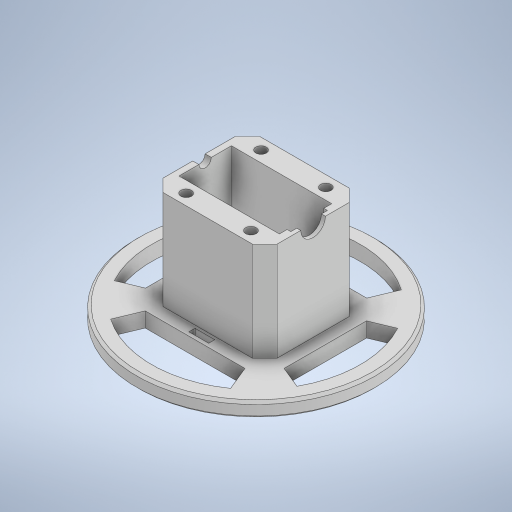
# Autodesk Inventor part: Base_baSECap
Saved by Autodesk Inventor 2023 (Build 270158000, 158)
## iProperties
Created: 2025-02-06
Part Number: Base_baSECap
Material: Generic
Document SubType Name: Modeling
Designer: Swoby
Density: 1 g/cm^3
Appearance: Default
Author: Swoby
Autodesk Inventor part; units mm, degrees
ref_plane "YZ Plane" through (0, 0, 0) normal (1, 0, 0) x (0, 1, 0)
ref_plane "XZ Plane" through (0, 0, 0) normal (0, 1, 0) x (-1, 0, 0)
ref_plane "XY Plane" through (0, 0, 0) normal (0, 0, 1) x (1, 0, 0)
sketch "Sketch1" plane through (0, 0, 0) normal (0, 0, 1) x (1, 0, 0)
  line L0 (0, 3) -> (0, -3)
  line L1 (0, 3) -> (47.2, 3)
  line L2 (48.2, 2) -> (48.2, -2)
  line L3 (47.2, -3) -> (0, -3)
  line L4 (0, 0) -> (48.2, 0) construction
  line L5 (47.2, 3) -> (48.2, 2)
  line L6 (48.2, -2) -> (47.2, -3)
  point P0 (48.2, 3)
  point P1 (48.2, -3)
  dimension "d0" = 96.4
  dimension "d1" = 6
  dimension "d2" = 1
  dimension "d3" = 1
  dimension "d4" = 1
  dimension "d5" = 1
  constraints: 14 end point, 4 point on line, 3 perpendicular, 2 midpoint, 1 horizontal, 1 vertical
  measures "d0" diameter of L2 L0
  measures "d1" distance of point (48.2, 3) point (48.2, -3)
  measures "d2" distance of L1.end point (48.2, 3)
  measures "d3" distance of L2.start point (48.2, 3)
  measures "d4" distance of L2.end point (48.2, -3)
  measures "d5" distance of L3.start point (48.2, -3)
revolve "Revolution1" add sketch "Sketch1" angle 360 about axis through (0, 3, 0) along (0, -1, 0)
sketch "Sketch2" plane through (0, -3, 0) normal (0, -1, 0) x (1, 0, 0)
  circle A0 centre (0, 0) radius 47.2 projected
  line L0 (0, 0) -> (47.2, 0) construction
  line L1 (0, 0) -> (12.9047, -12.9047) construction
  line L2 (0, 0) -> (-12.9047, -12.9047) construction
  arc A1 (11.7375, -14.5288) -> (14.3189, -14.3189) centre (12.9047, -12.9047) ccw
  arc A2 (-14.3189, -14.3189) -> (-11.7375, -14.5288) centre (-12.9047, -12.9047) ccw
  line L3 (4.5962, -4.5962) -> (1.8031, -7.3893) construction
  line L4 (-4.5962, -4.5962) -> (-1.8031, -7.3893) construction
  line L5 (12.9047, -12.9047) -> (14.3189, -14.3189) construction
  line L6 (-12.9047, -12.9047) -> (-14.3189, -14.3189) construction
  line L7 (-1.8031, -7.3893) -> (-11.7375, -14.5288)
  line L8 (1.8031, -7.3893) -> (11.7375, -14.5288)
  arc A3 (1.8031, -7.3893) -> (-1.8031, -7.3893) centre (0, -9.8982) ccw
  line L9 (4.5962, 4.5962) -> (7.3893, 1.8031) construction
  line L10 (7.3893, 1.8031) -> (14.5288, 11.7375)
  line L11 (12.9047, 12.9047) -> (14.3189, 14.3189) construction
  arc A4 (14.5288, 11.7375) -> (14.3189, 14.3189) centre (12.9047, 12.9047) ccw
  arc A5 (7.3893, 1.8031) -> (7.3893, -1.8031) centre (9.8982, 0) ccw
  line L12 (4.5962, -4.5962) -> (7.3893, -1.8031) construction
  line L13 (7.3893, -1.8031) -> (14.5288, -11.7375)
  arc A6 (14.3189, -14.3189) -> (14.5288, -11.7375) centre (12.9047, -12.9047) ccw
  line L14 (12.9047, -12.9047) -> (14.3189, -14.3189) construction
  line L15 (-4.5962, 4.5962) -> (-1.8031, 7.3893) construction
  line L16 (-1.8031, 7.3893) -> (-11.7375, 14.5288)
  line L17 (-12.9047, 12.9047) -> (-14.3189, 14.3189) construction
  arc A7 (-11.7375, 14.5288) -> (-14.3189, 14.3189) centre (-12.9047, 12.9047) ccw
  arc A8 (-1.8031, 7.3893) -> (1.8031, 7.3893) centre (0, 9.8982) ccw
  line L18 (4.5962, 4.5962) -> (1.8031, 7.3893) construction
  line L19 (1.8031, 7.3893) -> (11.7375, 14.5288)
  arc A9 (14.3189, 14.3189) -> (11.7375, 14.5288) centre (12.9047, 12.9047) ccw
  line L20 (12.9047, 12.9047) -> (14.3189, 14.3189) construction
  line L21 (-4.5962, -4.5962) -> (-7.3893, -1.8031) construction
  line L22 (-7.3893, -1.8031) -> (-14.5288, -11.7375)
  line L23 (-12.9047, -12.9047) -> (-14.3189, -14.3189) construction
  arc A10 (-14.5288, -11.7375) -> (-14.3189, -14.3189) centre (-12.9047, -12.9047) ccw
  arc A11 (-7.3893, -1.8031) -> (-7.3893, 1.8031) centre (-9.8982, 0) ccw
  line L24 (-4.5962, 4.5962) -> (-7.3893, 1.8031) construction
  line L25 (-7.3893, 1.8031) -> (-14.5288, 11.7375)
  arc A12 (-14.3189, 14.3189) -> (-14.5288, 11.7375) centre (-12.9047, 12.9047) ccw
  line L26 (-12.9047, 12.9047) -> (-14.3189, 14.3189) construction
  circle A13 centre (0, 0) radius 3.4
  point P0 (0, 0)
  dimension "d7" = 45
  dimension "d8" = 18.25
  dimension "d9" = 18.25
  dimension "d10" = 4
  dimension "d11" = 4
  dimension "d13" = 6.5
  dimension "d14" = 6.5
  dimension "d15" = 3.95
  dimension "d16" = 3.95
  dimension "d19" = 360
  dimension "d68" = 6.8
  constraints: 54 end point, 24 point on circle, 13 centre point, 9 coincident, 3 perpendicular, 3 tangent, 2 collinear, 2 point on line, 1 horizontal, 1 horizontal alignment, 90 other
  measures "d7" angle of L0 L1
  measures "d8" distance of L0.start L1.end
  measures "d9" distance of L0.start L2.end
  measures "d10" diameter of A1
  measures "d11" diameter of A2
  measures "d13" distance from line of point (0, 0) L3
  measures "d14" distance from line of point (0, 0) L4
  measures "d15" distance of L4.start L4.end
  measures "d16" distance of L3.start L3.end
  measures "d68" diameter of A13
extrude "Extrusion1" cut sketch "Sketch2" against normal blind 4 contours L8 A3 L7 A2 A10 L22 A11 L25 A12 A7 L16 A8 L19 A9 A4 L10 A5 L13 A6 A1 | A13
sketch "Sketch3" plane through (0, 1, 0) normal (0, -1, 0) x (1, 0, 0)
  arc A0 (11.7375, -14.5288) -> (14.5288, -11.7375) centre (12.9047, -12.9047) ccw projected
  line L0 (7.3893, -1.8031) -> (14.5288, -11.7375) projected
  arc A1 (7.3893, 1.8031) -> (7.3893, -1.8031) centre (9.8982, 0) ccw projected
  line L1 (14.5288, 11.7375) -> (7.3893, 1.8031) projected
  arc A2 (14.5288, 11.7375) -> (11.7375, 14.5288) centre (12.9047, 12.9047) ccw projected
  line L2 (1.8031, 7.3893) -> (11.7375, 14.5288) projected
  arc A3 (-1.8031, 7.3893) -> (1.8031, 7.3893) centre (0, 9.8982) ccw projected
  line L3 (-11.7375, 14.5288) -> (-1.8031, 7.3893) projected
  arc A4 (-11.7375, 14.5288) -> (-14.5288, 11.7375) centre (-12.9047, 12.9047) ccw projected
  line L4 (-7.3893, 1.8031) -> (-14.5288, 11.7375) projected
  arc A5 (-7.3893, -1.8031) -> (-7.3893, 1.8031) centre (-9.8982, 0) ccw projected
  line L5 (-14.5288, -11.7375) -> (-7.3893, -1.8031) projected
  arc A6 (-14.5288, -11.7375) -> (-11.7375, -14.5288) centre (-12.9047, -12.9047) ccw projected
  line L6 (-1.8031, -7.3893) -> (-11.7375, -14.5288) projected
  arc A7 (1.8031, -7.3893) -> (-1.8031, -7.3893) centre (0, -9.8982) ccw projected
  line L7 (11.7375, -14.5288) -> (1.8031, -7.3893) projected
  circle A8 centre (-12.9047, 12.9047) radius 0.5
  circle A9 centre (-12.9047, -12.9047) radius 0.5
  circle A10 centre (12.9047, -12.9047) radius 0.5
  circle A11 centre (12.9047, 12.9047) radius 0.5
  point P0 (0, 0)
  dimension "d23" = 1
  dimension "d24" = 1
  dimension "d25" = 1
  dimension "d26" = 1
  constraints: 4 centre point, 4 coincident
  measures "d23" diameter of A8
  measures "d24" diameter of A9
  measures "d25" diameter of A10
  measures "d26" diameter of A11
extrude "Extrusion2" cut sketch "Sketch3" against normal blind 6 contours A8 | A9 | A10 | A11
sketch "Sketch4" plane through (0, 3, 0) normal (0, 1, 0) x (1, 0, 0)
  line L0 (20, 10.65) -> (12.5, 10.65)
  line L1 (-20.6, 10.65) -> (-20.6, -10.55)
  line L2 (-20.6, -10.55) -> (8.8, -10.55)
  line L3 (20, -10.55) -> (20, 10.65)
  line L4 (21.5, 7.4) -> (20, 7.4)
  line L5 (20, 7.4) -> (20, 0)
  line L6 (21.5, 0) -> (21.5, 7.4)
  line L7 (23.1, 5) -> (21.5, 5)
  line L8 (21.5, 5) -> (21.5, 0)
  line L9 (20, 0) -> (23.1, 0)
  line L10 (23.1, 0) -> (23.1, 5)
  line L11 (8.8, 10.65) -> (12.5, 10.65)
  line L12 (8.8, -10.55) -> (12.5, -10.55)
  line L13 (-16.7, 10.65) -> (-11.3, 10.65)
  line L14 (-16.7, 10.65) -> (-20.6, 10.65)
  line L15 (-11.3, 10.65) -> (-16.7, 10.65)
  line L16 (12.5, 10.65) -> (12.5, 10.65)
  line L17 (8.8, 10.65) -> (-11.3, 10.65)
  line L18 (12.5, 10.65) -> (8.8, 10.65)
  line L19 (8.8, -10.55) -> (12.5, -10.55)
  line L20 (12.5, -10.55) -> (20, -10.55)
  line L21 (-23.1, 14.65) -> (-23.1, -14.55)
  line L22 (-18.1, 19.65) -> (18.1, 19.65)
  line L23 (23.1, 14.65) -> (23.1, -14.55)
  line L24 (18.1, -19.55) -> (-18.1, -19.55)
  line L25 (-23.1, -14.55) -> (-18.1, -19.55)
  line L26 (18.1, -19.55) -> (23.1, -14.55)
  line L27 (18.1, 19.65) -> (23.1, 14.65)
  line L28 (-18.1, 19.65) -> (-23.1, 14.65)
  line L29 (-23.1, 0) -> (23.1, 0) construction
  line L30 (8.8, 10.65) -> (8.8, -10.55)
  line L31 (12.5, -10.55) -> (12.5, 10.65)
  line L32 (-16.7, 10.65) -> (-16.7, -10.55) construction
  line L33 (-11.3, 10.65) -> (-11.3, -10.55) construction
  point P0 (0, 0)
  point P1 (-23.1, 19.65)
  point P2 (-23.1, -19.55)
  point P3 (-23.1, -2.3384)
  point P4 (23.1, 19.65)
  point P5 (23.1, -19.55)
  point P6 (-16.7, 19.65)
  point P7 (-11.3, 19.65)
  point P8 (0, 0)
  dimension "d29" = 10.65
  dimension "d30" = 1.5
  dimension "d31" = 1.6
  dimension "d32" = 21.2
  dimension "d33" = 40.6
  dimension "d40" = 2.5
  dimension "d41" = 5
  dimension "d47" = 5
  dimension "d48" = 5
  dimension "d49" = 5
  dimension "d50" = 5
  dimension "d51" = 5
  dimension "d52" = 5
  dimension "d53" = 5
  dimension "d54" = 5
  dimension "d57" = 7.4
  dimension "d77" = 3.7
  dimension "d78" = 7.5
  dimension "d79" = 3.9
  dimension "d80" = 5.4
  dimension "d81" = 9
  dimension "d82" = 9
  constraints: 68 end point, 21 parallel, 17 point on line, 12 horizontal, 11 perpendicular, 1 coincident, 1 collinear, 1 midpoint, 1 vertical
  measures "d29" distance from line of L5.end L0
  measures "d30" distance of L4.start L4.end
  measures "d31" distance of L7.start L7.end
  measures "d32" distance of L3.start L0.start
  measures "d33" distance between parallel lines of L3 L1
  measures "d40" distance from line of L1 point (-23.1, -2.338)
  measures "d41" distance between parallel lines of L9 L7
  measures "d47" distance of L21.end point (-23.1, -19.55)
  measures "d48" distance of L24.end point (-23.1, -19.55)
  measures "d49" distance of L24.start point (23.1, -19.55)
  measures "d50" distance of L23.end point (23.1, -19.55)
  measures "d51" distance of L22.end point (23.1, 19.65)
  measures "d52" distance of L23.start point (23.1, 19.65)
  measures "d53" distance of L22.start point (-23.1, 19.65)
  measures "d54" distance of L21.start point (-23.1, 19.65)
  measures "d57" distance between parallel lines of L9 L4
  measures "d77" distance between parallel lines of L30 L31
  measures "d78" distance between parallel lines of L3 L31
  measures "d79" distance between parallel lines of L32 L1
  measures "d80" distance between parallel lines of L33 L32
  measures "d81" distance between parallel lines of L17 L22
  measures "d82" distance between parallel lines of L24 L20
extrude "Extrusion3" add sketch "Sketch4" along normal blind 40
extrude "Extrusion5" cut sketch "Sketch4" against normal blind 30.95 from surface at 40 contours L3 L20 L31 L0 | L31 L12 L30 L11 | L30 L2 L1 L14 L13 L17
sketch "Sketch5" plane through (0, 43, 0) normal (0, 1, 0) x (1, 0, 0)
  line L0 (18.1, 19.65) -> (-18.1, 19.65) projected
  line L1 (-18.1, 19.65) -> (-23.1, 14.65) projected
  line L2 (-23.1, 14.65) -> (-23.1, -14.55) projected
  line L3 (-23.1, -14.55) -> (-18.1, -19.55) projected
  line L4 (-18.1, -19.55) -> (18.1, -19.55) projected
  line L5 (18.1, -19.55) -> (23.1, -14.55) projected
  line L6 (23.1, -14.55) -> (23.1, 14.65) projected
  line L7 (23.1, 14.65) -> (18.1, 19.65) projected
  line L8 (-20.6, 10.65) -> (20, 10.65) projected
  line L9 (20, 10.65) -> (20, -10.55) projected
  line L10 (20, -10.55) -> (-20.6, -10.55) projected
  line L11 (-20.6, -10.55) -> (-20.6, 10.65) projected
  line L12 (20, 7.4) -> (21.5, 7.4)
  line L13 (21.5, 7.4) -> (21.5, 5)
  line L14 (21.5, 5) -> (23.1, 5)
  line L15 (23.1, 5) -> (23.1, 0)
  line L16 (23.1, 0) -> (20, 0)
  line L17 (20, 7.4) -> (20, 0)
  line L18 (-23.1, 0) -> (-20.6, 0)
  line L19 (-20.6, 0) -> (-20.6, 2.5)
  line L20 (-20.6, 2.5) -> (-23.1, 2.5)
  line L21 (-23.1, 2.5) -> (-23.1, 0)
  point P0 (0, 0)
  point P1 (-21.85, 0)
  dimension "d62" = 10
  dimension "d63" = 14.8
  dimension "d64" = 1.5
  dimension "d66" = 5
  constraints: 20 end point, 8 point on line, 4 perpendicular, 2 horizontal, 2 parallel, 1 collinear, 1 midpoint
  measures "d62" diameter of L14 L16
  measures "d63" diameter of L12 L16
  measures "d64" distance of L12.start L12.end
  measures "d66" diameter of L20 point (-21.85, 0)
revolve "Revolution2" cut sketch "Sketch5" angle 360 about axis through (23.1, 43, 0) along (-1, 0, 0) contours L6 L16 L9 L12 L13 L14 | L20 L11 L18 L2
extrude "Extrusion6" cut sketch "Sketch2" against normal through all contours A13
sketch "Sketch6" plane through (0, 43, 0) normal (0, 1, 0) x (1, 0, 0)
  line L0 (21.5, 5) -> (23.1, 5) projected
  line L1 (23.1, 5) -> (23.1, 14.65) projected
  line L2 (23.1, 14.65) -> (18.1, 19.65) projected
  line L3 (18.1, 19.65) -> (-18.1, 19.65) projected
  line L4 (-18.1, 19.65) -> (-23.1, 14.65) projected
  line L5 (-23.1, 14.65) -> (-23.1, 2.5) projected
  line L6 (-23.1, 2.5) -> (-20.6, 2.5) projected
  line L7 (-20.6, 2.5) -> (-20.6, 10.65) projected
  line L8 (-20.6, 10.65) -> (20, 10.65) projected
  line L9 (20, 10.65) -> (20, 7.4) projected
  line L10 (20, 7.4) -> (21.5, 7.4) projected
  line L11 (21.5, 7.4) -> (21.5, 5) projected
  line L12 (23.1, -5) -> (21.5, -5) projected
  line L13 (21.5, -5) -> (21.5, -7.4) projected
  line L14 (21.5, -7.4) -> (20, -7.4) projected
  line L15 (20, -7.4) -> (20, -10.55) projected
  line L16 (20, -10.55) -> (-20.6, -10.55) projected
  line L17 (-20.6, -10.55) -> (-20.6, -2.5) projected
  line L18 (-20.6, -2.5) -> (-23.1, -2.5) projected
  line L19 (-23.1, -2.5) -> (-23.1, -14.55) projected
  line L20 (-23.1, -14.55) -> (-18.1, -19.55) projected
  line L21 (-18.1, -19.55) -> (18.1, -19.55) projected
  line L22 (18.1, -19.55) -> (23.1, -14.55) projected
  line L23 (23.1, -14.55) -> (23.1, -5) projected
  line L24 (-18.1, 19.65) -> (-18.1, 10.65) construction
  line L25 (-18.1, 15.15) -> (0, 15.15) construction
  circle A0 centre (-13.1, 15.15) radius 2.15
  line L26 (0, 19.65) -> (0, 0) construction
  circle A1 centre (0, 0) radius 3.4 projected
  line L27 (0, 0) -> (-23.1, 0) construction
  circle A2 centre (13.1, 15.15) radius 2.15
  line L28 (0, 0) -> (23.1, 0) construction
  circle A3 centre (-13.1, -15.15) radius 2.15
  circle A4 centre (13.1, -15.15) radius 2.15
  dimension "d83" = 4.3
  dimension "d84" = 5
  constraints: 10 end point, 4 centre point, 4 symmetric about line, 2 horizontal, 2 midpoint, 2 point on line, 1 coincident, 1 perpendicular, 1 vertical, 3 other
  measures "d83" diameter of A0
  measures "d84" distance from line of L24 A0.centre
extrude "Extrusion7" cut sketch "Sketch6" against normal blind 15 contours A0 | A2 | A3 | A4
extrude "Extrusion8" cut sketch "Sketch4" against normal blind 7.5 from surface at 9.05 contours L31 L12 L30 L11
chamfer "Chamfer1" distance 2 angle 45 2 edges at (12.5, 12.05, -0.05) (8.8, 12.05, -0.05)
sketch "Sketch7" plane through (0, 3, 0) normal (0, 1, 0) x (1, 0, 0)
  line L0 (23.1, 14.65) -> (23.1, -14.55) projected
  line L1 (23.1, -14.55) -> (18.1, -19.55) projected
  line L2 (18.1, -19.55) -> (-18.1, -19.55) projected
  line L3 (-18.1, -19.55) -> (-23.1, -14.55) projected
  line L4 (-23.1, -14.55) -> (-23.1, 14.65) projected
  line L5 (-23.1, 14.65) -> (-18.1, 19.65) projected
  line L6 (-18.1, 19.65) -> (18.1, 19.65) projected
  line L7 (18.1, 19.65) -> (23.1, 14.65) projected
  circle A0 centre (0, 0) radius 47.2 projected
  circle A1 centre (0, 0) radius 42.2
  line L8 (-28.1, 16.7211) -> (-28.1, -16.6211)
  line L9 (-28.1, -16.6211) -> (-20.1711, -24.55)
  line L10 (-20.1711, -24.55) -> (20.1711, -24.55)
  line L11 (20.1711, -24.55) -> (28.1, -16.6211)
  line L12 (28.1, -16.6211) -> (28.1, 16.7211)
  line L13 (28.1, 16.7211) -> (20.1711, 24.65)
  line L14 (20.1711, 24.65) -> (-20.1711, 24.65)
  line L15 (-20.1711, 24.65) -> (-28.1, 16.7211)
  line L16 (-28.1, 16.7211) -> (-36.949, 20.3865)
  line L17 (-20.1711, 24.65) -> (-24.2626, 34.5278)
  line L18 (-28.1, -16.6211) -> (-36.9939, -20.305)
  line L19 (20.1711, 24.65) -> (24.2626, 34.5278)
  line L20 (-4, 23.15) -> (4, 23.15)
  line L21 (4, 23.15) -> (4, 20.65)
  line L22 (4, 20.65) -> (-4, 20.65)
  line L23 (-4, 20.65) -> (-4, 23.15)
  line L24 (0, 23.15) -> (0, 24.65) construction
  point P0 (0, 0)
  dimension "d90" = 5
  dimension "d91" = 5
  dimension "d92" = 135
  dimension "d93" = 112.5
  dimension "d94" = 112.5
  dimension "d95" = 112.5
  dimension "d96" = 112.5
  dimension "d102" = 2.5
  dimension "d103" = 1.5
  dimension "d104" = 8
  constraints: 34 end point, 4 point on circle, 2 midpoint, 2 parallel, 2 perpendicular, 1 centre point, 1 horizontal, 7 other
  measures "d90" radial gap between concentric circles of A0 A1
  measures "d91" distance between parallel lines of L4 L8
  measures "d92" angle of L8 L15
  measures "d93" angle of L8 L16
  measures "d94" angle of L15 L17
  measures "d95" angle of L14 L19
  measures "d96" angle of L18 L8
  measures "d102" distance of L22.end L20.start
  measures "d103" distance of L24.start L24.end
  measures "d104" distance of L20.start L20.end
extrude "Extrusion9" cut sketch "Sketch7" against normal through all contours L19 L14 L17 A1 | A1 L16 L8 L18 | L20 L21 L22 L23
pattern_circular "Circular Pattern1" count 2 over 360 about axis through (0, -10, 0) along (0, 1, 0) of "Extrusion9"
equation "\"d3\" = d2"
equation "\"d4\" = d2"
equation "\"d5\" = d4"
equation "\"d9\" = d8"
equation "\"d48\" = d47"
equation "\"d49\" = d47"
equation "\"d50\" = d49"
equation "\"d51\" = d47"
equation "\"d52\" = d51"
equation "\"d53\" = d47"
equation "\"d54\" = d53"
equation "\"d94\" = d93"
equation "\"d95\" = d93"
equation "\"d96\" = d93"
body "Solid1"
